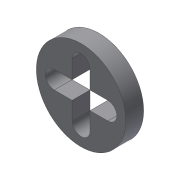
# Autodesk Inventor part: lid
Saved by Autodesk Inventor 2018 (Build 220112000, 112)
## iProperties
Created: 2020-03-26
Part Number: lid
Material: Generic
Document SubType Name: Modeling
Designer: Matt
Density: 1 g/cm^3
Appearance: Default
Author: Matt
Autodesk Inventor part; units mm, degrees
ref_plane "YZ Plane" through (0, 0, 0) normal (1, 0, 0) x (0, 1, 0)
ref_plane "XZ Plane" through (0, 0, 0) normal (0, 1, 0) x (-1, 0, 0)
ref_plane "XY Plane" through (0, 0, 0) normal (0, 0, 1) x (1, 0, 0)
sketch "Sketch1" plane through (0, 0, 0) normal (0, 0, 1) x (1, 0, 0)
  circle A0 centre (0, 0) radius 15.875 projected
extrude "Extrusion1" add sketch "Sketch1" along normal blind 6.35
sketch "Sketch2" plane through (0, 0, 6.35) normal (0, 0, 1) x (1, 0, 0)
  arc A0 (3.175, 9.525) -> (-3.175, 9.525) centre (0, 9.525) ccw projected
  line L0 (3.175, 9.525) -> (3.175, 3.175) projected
  line L1 (3.175, 3.175) -> (9.525, 3.175) projected
  arc A1 (9.525, -3.175) -> (9.525, 3.175) centre (9.525, 0) ccw projected
  line L2 (9.525, -3.175) -> (3.175, -3.175) projected
  line L3 (3.175, -3.175) -> (3.175, -9.525) projected
  arc A2 (-3.175, -9.525) -> (3.175, -9.525) centre (0, -9.525) ccw projected
  line L4 (-3.175, -9.525) -> (-3.175, -3.175) projected
  line L5 (-3.175, -3.175) -> (-9.525, -3.175) projected
  arc A3 (-9.525, 3.175) -> (-9.525, -3.175) centre (-9.525, 0) ccw projected
  line L6 (-9.525, 3.175) -> (-3.175, 3.175) projected
  line L7 (-3.175, 3.175) -> (-3.175, 9.525) projected
  circle A4 centre (0, 0) radius 15.875 projected
extrude "Extrusion2" cut sketch "Sketch2" against normal through all contours L0 L1 A1 L2 L3 A2 L4 L5 A3 L6 L7 A0
body "Solid1"
